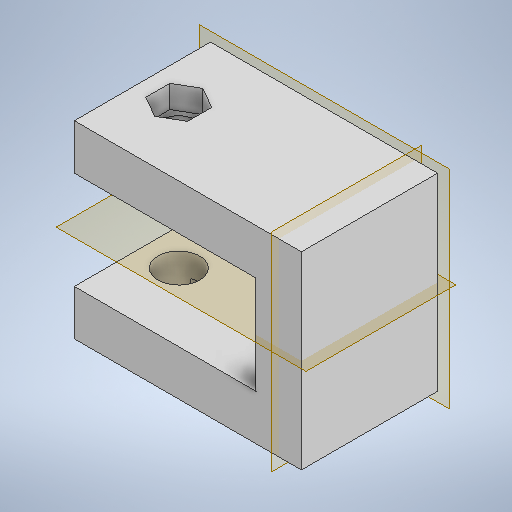
# Autodesk Inventor part: PruebaCParaBuje
Saved by Autodesk Inventor 2025.2 (Build 292293000, 293)
## iProperties
Created: 2025-04-03
Part Number: PruebaCParaBuje
Material: Genérico
Document SubType Name: Modeling
Designer: braug
Density: 1 g/cm^3
Appearance: Valor por defecto
Author: braug
Autodesk Inventor part; units mm, degrees
sketch "Boceto1" plane through (0, 0, 0) normal (0, 0, 1) x (1, 0, 0)
  line L0 (-2.5, -10.4) -> (2.5, -10.4)
  line L1 (2.5, -10.4) -> (2.5, 10.4)
  line L2 (2.5, 10.4) -> (-2.5, 10.4)
  line L3 (-2.5, 5.4) -> (-2.5, -5.4)
  line L4 (-2.5, -10.4) -> (2.5, 10.4) construction
  line L5 (2.5, -10.4) -> (-2.5, 10.4) construction
  line L6 (-2.5, 10.4) -> (-22.5, 10.4)
  line L7 (-22.5, 10.4) -> (-22.5, 5.4)
  line L8 (-22.5, 5.4) -> (-2.5, 5.4)
  line L9 (-27.5, 0) -> (7.5, 0) projected
  line L10 (-2.5, -10.4) -> (-22.5, -10.4)
  line L11 (-22.5, -10.4) -> (-22.5, -5.4)
  line L12 (-22.5, -5.4) -> (-2.5, -5.4)
  point P0 (0, 0)
  dimension "d4" = 25
  dimension "d5" = 20
  dimension "d6" = 10.8
  dimension "d8" = 20.8
  constraints: 24 end point, 3 parallel, 3 symmetric about line, 2 horizontal, 2 midpoint, 2 perpendicular
  measures "d4" distance of L1.end L6.end
  measures "d5" distance of L3.start L7.end
  measures "d6" distance of L12.start L7.end
  measures "d8" distance of L0.end L1.end
extrude "Extrusión1" add sketch "Boceto1" along normal blind 15
sketch "Boceto2" plane through (-22.5, -10.4, 0) normal (0, -1, 0) x (1, 0, 0)
  line L0 (0, 0) -> (0, 15) projected
  line L1 (0, 15) -> (25, 15) projected
  line L2 (2, 12.5) -> (6, 12.5)
  line L3 (6, 2.5) -> (2, 2.5)
  line L4 (2, 12.5) -> (6, 2.5) construction
  line L5 (6, 12.5) -> (2, 2.5) construction
  line L6 (4.8542, 9.6355) -> (6, 12.5)
  line L7 (3.1458, 9.6355) -> (2, 12.5)
  line L8 (3.1458, 5.3645) -> (2, 2.5)
  line L9 (4.8542, 5.3645) -> (6, 2.5)
  arc A0 (4.8542, 5.3645) -> (4.8542, 9.6355) centre (4, 7.5) ccw
  arc A1 (3.1458, 9.6355) -> (3.1458, 5.3645) centre (4, 7.5) ccw
  point P0 (22.5, 0)
  point P1 (0, 7.5)
  dimension "d11" = 4
  dimension "d13" = 7.5
  dimension "d25" = 2.3
  dimension "d26" = 2.3
  constraints: 16 end point, 4 collinear, 4 point on circle, 4 point on line, 3 midpoint, 2 centre point, 1 horizontal, 1 parallel
  measures "d11" distance of A0.centre point (0, 7.5)
  measures "d13" distance from line of L1 A0.centre
  measures "d25" radius of A0
  measures "d26" radius of A1
extrude "Extrusión2" cut sketch "Boceto2" against normal blind 2.5
sketch "Boceto3" plane through (-22.5, -7.9, 0) normal (0, -1, 0) x (1, 0, 0)
  arc A0 (4.8542, 5.3645) -> (4.8542, 9.6355) centre (4, 7.5) ccw projected
  arc A1 (3.1458, 9.6355) -> (3.1458, 5.3645) centre (4, 7.5) ccw projected
  circle A2 centre (4, 7.5) radius 2.3
  point P0 (22.5, 0)
  point P1 (3.1458, 5.3645)
  point P2 (4.8542, 5.3645)
  point P3 (4.8542, 9.6355)
  point P4 (3.1458, 9.6355)
  dimension "d27" = 4.6
  constraints: 1 centre point, 1 coincident
  measures "d27" diameter of A2
extrude "Extrusión3" cut sketch "Boceto3" against normal blind 2.5
sketch "Boceto4" plane through (-22.5, 10.4, 0) normal (0, 1, 0) x (1, 0, 0)
  circle A0 centre (4, -7.5) radius 2.3 construction
  line L0 (6.3, -8.8279) -> (4, -10.1558)
  line L1 (4, -10.1558) -> (1.7, -8.8279)
  line L2 (1.7, -8.8279) -> (1.7, -6.1721)
  line L3 (1.7, -6.1721) -> (4, -4.8442)
  line L4 (4, -4.8442) -> (6.3, -6.1721)
  line L5 (6.3, -6.1721) -> (6.3, -8.8279)
  point P0 (22.5, 0)
  point P1 (6.3, -7.5)
  constraints: 12 end point, 1 coincident, 1 horizontal alignment, 1 midpoint, 14 other
extrude "Extrusión4" cut sketch "Boceto4" against normal blind 2.5
sketch "Boceto5" plane through (-22.5, 7.9, 0) normal (0, 1, 0) x (1, 0, 0)
  arc A0 (4.8542, -9.6355) -> (4.8542, -5.3645) centre (4, -7.5) ccw projected
  circle A1 centre (4, -7.5) radius 1.75
  point P0 (22.5, 0)
  point P1 (3.1458, -5.3645)
  point P2 (3.1458, -9.6355)
  dimension "d22" = 3.5
  constraints: 1 centre point, 1 coincident
  measures "d22" diameter of A1
extrude "Extrusión5" cut sketch "Boceto5" against normal blind 2.5
